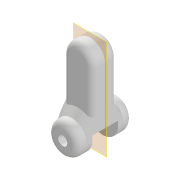
# Autodesk Inventor part: middle_f3
Saved by Autodesk Inventor 2020.2 (Build 242310000, 310)
## iProperties
Created: 2020-04-08
Part Number: middle_f3
Material: Generic
Document SubType Name: Modeling
Designer: Bardo91
Density: 1 g/cm^3
Appearance: Default
Author: Bardo91
Autodesk Inventor part; units mm, degrees
ref_plane "YZ Plane" through (0, 0, 0) normal (1, 0, 0) x (0, 1, 0)
ref_plane "XZ Plane" through (0, 0, 0) normal (0, 1, 0) x (-1, 0, 0)
ref_plane "XY Plane" through (0, 0, 0) normal (0, 0, 1) x (1, 0, 0)
sketch "Sketch1" plane through (0, 0, 0) normal (0, 0, 1) x (1, 0, 0)
  circle A0 centre (0, 0) radius 1.5
  circle A1 centre (0, 0) radius 5
  line L0 (0, 0) -> (0, 20)
  circle A2 centre (0, 20) radius 1.5
  circle A3 centre (0, 20) radius 5
  line L1 (-5, 20) -> (-5, 0)
  line L2 (5, 0) -> (5, 20)
  dimension "d0" = 3
  dimension "d1" = 10
  dimension "d2" = 20
  dimension "d3" = 3
  dimension "d4" = 10
  constraints: 6 end point, 4 centre point, 4 coincident, 4 point on circle, 3 tangent, 1 vertical
  measures "d0" diameter of A0
  measures "d1" diameter of A1
  measures "d2" distance of L0.start L0.end
  measures "d3" diameter of A2
  measures "d4" diameter of A3
extrude "Extrusion1" add sketch "Sketch1" along normal blind 8 contours A1 | L1 A3 L0 A1 | A1 L0 A3 L2 | A3 | A2
sketch "Sketch2" plane through (0, 0, 8) normal (0, 0, 1) x (1, 0, 0)
  circle A0 centre (0, 0) radius 1.5
  circle A1 centre (0, 0) radius 5
  dimension "d7" = 3
  dimension "d8" = 10
  constraints: 2 centre point, 2 coincident
  measures "d7" diameter of A0
  measures "d8" diameter of A1
extrude "Extrusion2" add sketch "Sketch2" along normal blind 5
ref_plane "Work Plane1" through (0, 0, 4) normal (0, 0, 1) x (1, 0, 0)
mirror "Mirror1" about plane through (0, 0, 4) normal (0, 0, 1) of "Extrusion2"
chamfer "Chamfer1" distance 2 angle 45 2 edges at (0, 5, 0) (0, 5, 8)
fillet "Fillet1" radius 2 8 edges at (-5, 0, 13) (0, 25, 8) (-5, 12.4495, 8) (5, 12.4495, 8) (0, 25, 0) (-5, 12.4495, 0) (5, 12.4495, 0) (-5, 0, -5)
sketch "Sketch3" plane through (0, 0, 4) normal (0, 0, 1) x (1, 0, 0)
  circle A0 centre (0, 0) radius 5.25
  line L0 (0, 0) -> (-10, 0)
  line L1 (-10, 0) -> (-10, 5.25)
  line L2 (-10, 5.25) -> (0, 5.25)
  line L3 (0, 0) -> (0, 5.25)
  point P0 (-5.25, 0)
  dimension "d15" = 10.5
  dimension "d21" = 10
  dimension "d22" = 5.25
  constraints: 8 end point, 2 horizontal, 2 perpendicular, 1 coincident, 3 other
  measures "d21" distance of L0.start L0.end
  measures "d22" distance of L0.end L1.end
extrude "Extrusion3" cut sketch "Sketch3" along normal mid plane 8.5
sketch "Sketch4" plane through (0, 0, 4) normal (0, 0, 1) x (1, 0, 0)
  line L0 (5, 7.4833) -> (5, 20) projected
  line L1 (5, 7.4833) -> (5.9039, 5)
  line L2 (5, 7.4833) -> (7.6427, 7.4833) construction
  line L3 (5.9039, 5) -> (5.9039, 0)
  line L4 (5.9039, 0) -> (5, 0)
  line L5 (5, 0) -> (5, 7.4833)
  point P0 (0, 0)
  dimension "d18" = 70
  constraints: 10 end point, 2 perpendicular, 1 equal length, 1 horizontal, 1 parallel, 1 point on line
  measures "d18" angle of L1 L2
extrude "Extrusion4" add sketch "Sketch4" along normal mid plane 5
body "Solid1"
